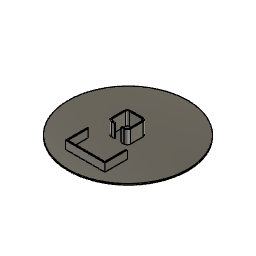
步进电机支架 v3 (Autodesk Fusion 360 design; units mm, degrees)
Autodesk Fusion 360 part; units mm, degrees
sketch "草图1" plane through (0, 0, 0) normal (0, 0, 1) x (1, 0, 0)
  line L0 (-45, 25) -> (-12.9, 25)
  line L1 (-50, 20) -> (-50, -12.1)
  line L2 (-45, -17.1) -> (-12.9, -17.1)
  line L3 (-7.9, 20) -> (-7.9, -12.1)
  arc A0 (-50, -12.1) -> (-45, -17.1) centre (-45, -12.1) ccw
  arc A1 (-45, 25) -> (-50, 20) centre (-45, 20) ccw
  arc A2 (-7.9, 20) -> (-12.9, 25) centre (-12.9, 20) ccw
  arc A3 (-12.9, -17.1) -> (-7.9, -12.1) centre (-12.9, -12.1) ccw
  line L4 (-28.95, -17.1) -> (-28.95, 3.95)
  line L5 (-28.95, 3.95) -> (-7.9, 3.95)
  line L6 (-28.95, 3.95) -> (-7.9, 3.95)
  line L7 (-28.95, 3.95) -> (-50, 3.95)
  line L8 (-28.95, 3.95) -> (-28.95, 25)
  line L9 (-158.95, 3.95) -> (-28.95, -126.05)
  line L10 (-28.95, -126.05) -> (101.05, 3.95)
  line L11 (101.05, 3.95) -> (-28.95, 133.95)
  line L12 (-28.95, 133.95) -> (-158.95, 3.95)
  point P0 (-50, 25)
  point P1 (-7.9, 25)
  point P2 (-50, -17.1)
  dimension "d1" = 42.1
  dimension "d2" = 42.1
  dimension "d3" = 5
  dimension "d5" = 130
  dimension "d6" = 130
  dimension "d7" = 130
  dimension "d8" = 130
  constraint horizontal L0
  constraint perpendicular L0 L1
  constraint perpendicular L1 L2
  constraint perpendicular L2 L3
  constraint coincident P2 L1
  constraint coincident P2 L2
  constraint tangent L1 A0
  constraint tangent L2 A0
  constraint coincident P0 L1
  constraint coincident P0 L0
  constraint tangent L1 A1
  constraint tangent L0 A1
  constraint equal A0 A1
  constraint coincident P1 L0
  constraint coincident P1 L3
  constraint tangent L0 A2
  constraint tangent L3 A2
  constraint equal A0 A2
  constraint tangent L3 A3
  constraint tangent L2 A3
  constraint equal A0 A3
  constraint midpoint L3 L5.end
  constraint midpoint L1 L7.end
  constraint midpoint L2 L4.start
  constraint midpoint L0 L8.end
  constraint perpendicular L3 L5
  constraint perpendicular L4 L7
  constraint perpendicular L0 L8
  constraint perpendicular L9 L10
  measures "d1" distance of P0 P1
  measures "d2" distance of P0 P2
  measures "d3" radius of A0
  measures "d5" distance of L4.end L10.end
  measures "d6" distance of L4.end L9.start
  measures "d7" distance of L4.end L9.end
  measures "d8" distance of L4.end L11.end
extrude "拉伸1" add sketch "草图1" against normal blind 3 contours L0 L1 A1 L7 L8 | L0 L3 A2 L5 L6 L8 | L2 L3 A3 L4 L5 L6 | L1 L2 A0 L4 L7 | L9 L10 L11 L12 makes body 1
sketch "草图2" plane through (0, 0, 0) normal (0, 0, 1) x (-1, 0, 0)
  line L0 (28.95, -133.95) -> (158.95, -3.95)
  line L1 (158.95, -3.95) -> (28.95, 126.05)
  line L2 (28.95, 126.05) -> (-101.05, -3.95)
  line L3 (-101.05, -3.95) -> (28.95, -133.95)
  line L4 (45, -25) -> (13, -25)
  line L5 (8, -20) -> (8, 12)
  line L6 (45, 17) -> (13, 17)
  line L7 (50, -20) -> (50, 12)
  arc A0 (45, -25) -> (50, -20) centre (45, -20) ccw
  arc A1 (50, 12) -> (45, 17) centre (45, 12) ccw
  arc A2 (13, 17) -> (8, 12) centre (13, 12) ccw
  arc A3 (8, -20) -> (13, -25) centre (13, -20) ccw
  line L8 (45, 20) -> (13, 20)
  arc A4 (13, 20) -> (5, 12) centre (13, 12) ccw
  line L9 (5, -20) -> (5, 12)
  arc A5 (5, -20) -> (13, -28) centre (13, -20) ccw
  line L10 (45, -28) -> (13, -28)
  arc A6 (45, -28) -> (53, -20) centre (45, -20) ccw
  line L11 (53, -20) -> (53, 12)
  arc A7 (53, 12) -> (45, 20) centre (45, 12) ccw
  dimension "d12" = 5
  dimension "d13" = 3
  constraint horizontal L4
  constraint perpendicular L4 L5
  constraint perpendicular L5 L6
  constraint perpendicular L6 L7
  constraint tangent L4 A0
  constraint tangent L7 A0
  constraint tangent L6 A1
  constraint tangent L7 A1
  constraint equal A0 A1
  constraint tangent L6 A2
  constraint tangent L5 A2
  constraint equal A0 A2
  constraint tangent L5 A3
  constraint tangent L4 A3
  constraint equal A0 A3
  measures "d12" radius of A0
extrude "拉伸2" add sketch "草图2" along normal blind 15 contours L8 A4 L9 A5 L10 A6 L11 A7 bodies 1
sketch "草图3" plane through (0, 0, 15) normal (0, 0, 1) x (-1, 0, 0)
  arc A0 (45, -25) -> (50, -20) centre (45, -20) ccw
  line L0 (45, -25) -> (13, -25)
  arc A1 (8, -20) -> (13, -25) centre (13, -20) ccw
  line L1 (8, -20) -> (8, 12)
  arc A2 (13, 17) -> (8, 12) centre (13, 12) ccw
  line L2 (13, 17) -> (45, 17)
  arc A3 (50, 12) -> (45, 17) centre (45, 12) ccw
  line L3 (50, 12) -> (50, -20)
  arc A4 (45, -28) -> (53, -20) centre (45, -20) ccw
  line L4 (53, -20) -> (53, 12)
  arc A5 (53, 12) -> (45, 20) centre (45, 12) ccw
  line L5 (45, 20) -> (13, 20)
  arc A6 (13, 20) -> (5, 12) centre (13, 12) ccw
  line L6 (5, 12) -> (5, -20)
  arc A7 (5, -20) -> (13, -28) centre (13, -20) ccw
  line L7 (13, -28) -> (45, -28)
  line L8 (29, 20) -> (20.8, 20)
  line L9 (20.8, 20) -> (20.8, 17)
  line L10 (20.8, 17) -> (29, 17)
  line L11 (29, 17) -> (29, 20)
  line L12 (29, 20) -> (37.2, 20)
  line L13 (37.2, 20) -> (37.2, 17)
  line L14 (37.2, 17) -> (29, 17)
  line L15 (29, 17) -> (29, 20)
  dimension "d16" = 8.2
  constraint horizontal L8
  constraint vertical L9
  constraint horizontal L10
  constraint vertical L11
  constraint midpoint L5 L8.start
  constraint horizontal L12
  constraint vertical L13
  constraint horizontal L14
  constraint vertical L15
  measures "d16" distance of L8.start L8.end
extrude "拉伸3" cut sketch "草图3" against normal blind 15 contours L2 L5 L11 L12 L13 L14 L15 | L2 L5 L8 L9 L10 L11 L15 bodies 1
sketch "草图4" plane through (0, 0, 15) normal (0, 0, 1) x (-1, 0, 0)
  line L0 (20.8, 17) -> (20.8, 20)
  line L1 (20.8, 20) -> (13, 20)
  arc A0 (13, 20) -> (5, 12) centre (13, 12) ccw
  line L2 (5, 12) -> (5, -20)
  arc A1 (5, -20) -> (13, -28) centre (13, -20) ccw
  line L3 (13, -28) -> (45, -28)
  arc A2 (45, -28) -> (53, -20) centre (45, -20) ccw
  line L4 (53, -20) -> (53, 12)
  arc A3 (53, 12) -> (45, 20) centre (45, 12) ccw
  line L5 (45, 20) -> (37.2, 20)
  line L6 (37.2, 20) -> (37.2, 17)
  line L7 (37.2, 17) -> (45, 17)
  arc A4 (50, 12) -> (45, 17) centre (45, 12) ccw
  line L8 (50, 12) -> (50, -20)
  arc A5 (45, -25) -> (50, -20) centre (45, -20) ccw
  line L9 (45, -25) -> (13, -25)
  arc A6 (8, -20) -> (13, -25) centre (13, -20) ccw
  line L10 (8, -20) -> (8, 12)
  arc A7 (13, 17) -> (8, 12) centre (13, 12) ccw
  line L11 (13, 17) -> (20.8, 17)
extrude "拉伸4" add sketch "草图3" along normal blind 18 contours A0 L0 A1 L1 A2 L2 A3 L3 A4 L4 A5 L5 A6 L6 A7 L7 L9 L13 bodies 1
extrude "拉伸5" cut 1 faces at (21.4463, -46.7153, 0) along direction (0, 0, -1) blind 80 on bodies 1 bodies 1
sketch "草图5" plane through (0, 0, 0) normal (1, 0, 0) x (0, 1, 0)
sketch "草图6" plane through (0, 0, 0) normal (0, 0, 1) x (1, 0, 0)
  line L0 (-30, -20) -> (-90, -20)
  line L1 (-90, -20) -> (-90, 73.535)
  line L2 (-30, -20) -> (30, -20)
  line L3 (30, -20) -> (30, 73.535)
  line L4 (-30, 210.003) -> (-30, 210)
  line L5 (-90, 73.535) -> (30, 73.535)
  dimension "d23" = 60
  constraint horizontal L0
  constraint vertical L1
  constraint horizontal L2
  constraint vertical L3
  constraint vertical L4
  constraint perpendicular L3 L5
  measures "d23" distance of L0.start L2.end
sketch "草图7" plane through (0, 0, 0) normal (0, 0, 1) x (1, 0, 0)
move_body "移动1" bodies 1 to x (1, 0, 0) y (0, 1, 0) z (0, 0, 1) at (-196.9406, 20.0173, 0)
sketch "草图8" plane through (0, 0, 0) normal (0, 0, 1) x (1, 0, 0)
  line L0 (-217.7406, 0.0173) -> (-209.9406, 0.0173)
  arc A0 (-209.9406, 0.0173) -> (-201.9406, 8.0173) centre (-209.9406, 8.0173) ccw
  line L1 (-201.9406, 8.0173) -> (-201.9406, 40.0173)
  arc A1 (-201.9406, 40.0173) -> (-209.9406, 48.0173) centre (-209.9406, 40.0173) ccw
  line L2 (-209.9406, 48.0173) -> (-241.9406, 48.0173)
  arc A2 (-241.9406, 48.0173) -> (-249.9406, 40.0173) centre (-241.9406, 40.0173) ccw
  line L3 (-249.9406, 40.0173) -> (-249.9406, 8.0173)
  arc A3 (-249.9406, 8.0173) -> (-241.9406, 0.0173) centre (-241.9406, 8.0173) ccw
  line L4 (-241.9406, 0.0173) -> (-234.1406, 0.0173)
  line L5 (-234.1406, 0.0173) -> (-234.1406, 3.0173)
  line L6 (-234.1406, 3.0173) -> (-241.9406, 3.0173)
  arc A4 (-246.9406, 8.0173) -> (-241.9406, 3.0173) centre (-241.9406, 8.0173) ccw
  line L7 (-246.9406, 8.0173) -> (-246.9406, 40.0173)
  arc A5 (-241.9406, 45.0173) -> (-246.9406, 40.0173) centre (-241.9406, 40.0173) ccw
  line L8 (-241.9406, 45.0173) -> (-209.9406, 45.0173)
  arc A6 (-204.9406, 40.0173) -> (-209.9406, 45.0173) centre (-209.9406, 40.0173) ccw
  line L9 (-204.9406, 40.0173) -> (-204.9406, 8.0173)
  arc A7 (-209.9406, 3.0173) -> (-204.9406, 8.0173) centre (-209.9406, 8.0173) ccw
  line L10 (-209.9406, 3.0173) -> (-217.7406, 3.0173)
  line L11 (-217.7406, 3.0173) -> (-217.7406, 0.0173)
  circle A8 centre (-225, 25) radius 150
  line L12 (-178.0547, -28.4802) -> (-178.0547, -84.9802)
  line L13 (-178.0547, -84.9802) -> (-276.6987, -84.9802)
  line L14 (-276.6987, -84.9802) -> (-276.6987, -28.4802)
  line L15 (-276.6987, -28.4802) -> (-178.0547, -28.4802)
  line L16 (-273.6987, -81.9802) -> (-273.6987, -31.4802)
  line L17 (-273.6987, -31.4802) -> (-181.0547, -31.4802)
  line L18 (-181.0547, -31.4802) -> (-181.0547, -81.9802)
  line L19 (-181.0547, -81.9802) -> (-273.6987, -81.9802)
  line L20 (-273.6987, -31.4802) -> (-276.6987, -28.4802)
  line L21 (-181.0547, -31.4802) -> (-178.0547, -28.4802)
  dimension "d24" = 300
  dimension "d25" = 56.5
  constraint perpendicular L20 L21
  measures "d24" diameter of A8
  measures "d25" distance of L12.start L12.end
extrude "拉伸6" add sketch "草图8" against normal blind 3 contours A8 | L15 L17 L20 L21 | L12 L13 L14 L16 L18 L19 L20 L21 | L16 L17 L18 L19 bodies 1
extrude "拉伸7" add sketch "草图8" along normal blind 20 contours L12 L13 L14 L16 L18 L19 L20 L21 bodies 1
split "分割1" by plane through (0, 0, 0) normal (0, 0, 1) bodies 1 makes body 2 at (-231.274, 45.0173, 22) makes body 3 at (-210.936, -84.9802, 6.6667)
move_body "移动2" bodies 3 to x (1, 0, 0) y (0, 1, 0) z (0, 0, 1) at (5, 0, 0)
combine "合并1" operation add target body 2 tool bodies 3 1
